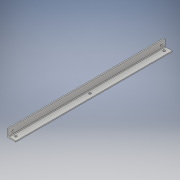
# Autodesk Inventor part: Part2
Saved by Autodesk Inventor 2017 (Build 210142000, 142)
## iProperties
Created: 2018-10-17
Part Number: Part2
Material: Generic
Document SubType Name: Modeling
Designer: ddeboer
Density: 1 g/cm^3
Appearance: Default
Author: ddeboer
Autodesk Inventor part; units mm, degrees
ref_plane "YZ Plane" through (0, 0, 0) normal (1, 0, 0) x (0, 1, 0)
ref_plane "XZ Plane" through (0, 0, 0) normal (0, 1, 0) x (-1, 0, 0)
ref_plane "XY Plane" through (0, 0, 0) normal (0, 0, 1) x (1, 0, 0)
sketch "Sketch1" plane through (0, 0, 0) normal (0, 0, 1) x (1, 0, 0)
  line L0 (0, 25.4) -> (0, 0)
  line L1 (0, 0) -> (25.4, 0)
  line L2 (3.175, 25.4) -> (3.175, 4.953)
  line L3 (4.953, 3.175) -> (25.4, 3.175)
  line L4 (0, 25.4) -> (3.175, 25.4)
  line L5 (25.4, 3.175) -> (25.4, 0)
  arc A0 (3.175, 4.953) -> (4.953, 3.175) centre (4.953, 4.953) ccw
  point P0 (3.175, 3.175)
  dimension "d0" = 25.4
  dimension "d1" = 25.4
  dimension "d2" = 3.175
  dimension "d21" = 1.778
  constraints: 14 end point, 2 perpendicular, 2 point on circle, 2 point on line, 2 tangent, 2 vertical, 1 centre point, 1 horizontal, 1 other
  measures "d0" distance of L0.start L0.end
  measures "d1" distance of L0.end L1.end
  measures "d2" distance between parallel lines of L2 L0
  measures "d21" radius of A0
extrude "Extrusion1" add sketch "Sketch1" along normal blind 492.125
sketch "Sketch2" plane through (3.175, 3.175, 0) normal (0, 1, 0) x (1, 0, 0)
  circle A0 centre (9.525, -479.425) radius 2.8398
  line L0 (22.225, -492.125) -> (1.778, -492.125) projected
  line L1 (22.225, 0) -> (22.225, -492.125) projected
  circle A1 centre (9.525, -12.7) radius 2.8398
  line L2 (22.225, 0) -> (1.778, 0) projected
  point P0 (-3.175, 0)
  point P1 (0, -501.65)
  point P2 (1.778, -492.125)
  dimension "d5" = 12.7
  dimension "d6" = 12.7
  dimension "d9" = 466.725
  dimension "d31" = 12.7
  constraints: 2 centre point, 1 vertical, 3 other
  measures "d6" distance from line of A0.centre L1
  measures "d9" distance of A0.centre A1.centre
  measures "d31" distance from line of A1.centre L2
hole "Hole1" at (12.7, 3.175, 479.425) at (12.7, 3.175, 12.7) direction (0, -1, 0) diameter 7.1374 depth 25.4 tip angle 118 clearance for "Flat Head Machine Screw (82)" size "1/4" standard "Ansi Unified Screw Threads"
sketch "Sketch5" plane through (4.953, 3.175, 0) normal (0, 1, 0) x (1, 0, 0)
  circle A0 centre (7.747, -479.425) radius 3.5687 projected
  circle A1 centre (7.747, -12.7) radius 3.5687 projected
  line L0 (7.747, -479.425) -> (7.747, -12.7) construction
  circle A2 centre (7.747, -246.0625) radius 2.5527
  point P0 (-4.953, 0)
  constraints: 2 end point, 1 centre point, 1 midpoint, 1 vertical
hole "Hole2" at (12.7, 3.175, 246.0625) direction (0, -1, 0) diameter 7.1374 depth 25.4 tip angle 118 clearance for "Flat Head Machine Screw (82)" size "1/4" standard "Ansi Unified Screw Threads"
sketch "Sketch6" plane through (3.175, 4.953, 0) normal (1, 0, 0) x (0, 0, -1)
  circle A0 centre (-479.425, 7.747) radius 3.2153
  line L0 (-492.125, 0) -> (-492.125, 20.447) projected
  line L1 (0, 20.447) -> (-492.125, 20.447) projected
  circle A1 centre (-12.7, 7.747) radius 3.3329
  point P0 (0, -4.953)
  dimension "d32" = 12.7
  dimension "d33" = 12.7
  dimension "d34" = 466.725
  dimension "d35" = 12.7
  constraints: 2 centre point
  measures "d32" distance from line of A0.centre L0
  measures "d33" distance from line of A0.centre L1
  measures "d34" distance of A1.centre A0.centre
  measures "d35" distance from line of A1.centre L1
hole "Hole3" at (3.175, 12.7, 479.425) at (3.175, 12.7, 12.7) direction (-1, 0, 0) diameter 7.1374 depth 25.4 tip angle 118 clearance for "Flat Head Machine Screw (82)" size "1/4" standard "Ansi Unified Screw Threads"
body "Solid1"
